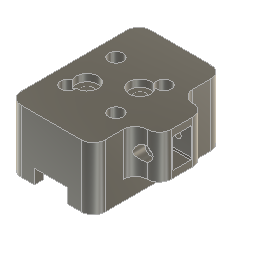
XY Bracket Bottom (Autodesk Fusion 360 archive; units mm, degrees)
design "XY Bracket Bottom Left"
part number: XY Brackets
part number: Left Bottom
Autodesk Fusion 360 part; units mm, degrees
sketch "Sketch1" plane through (0, 0, 0) normal (0, 0, 1) x (1, 0, 0) in component "Left Bottom"
  line L0 (27, -17.5) -> (-27, -17.5)
  line L1 (-27, -17.5) -> (-27, 17.5)
  line L2 (-27, 17.5) -> (27, 17.5)
  line L3 (27, 17.5) -> (27, -17.5)
  line L4 (27, -17.5) -> (-27, 17.5) construction
  line L5 (-27, -17.5) -> (27, 17.5) construction
  line L6 (23, 13.5) -> (-23, 13.5)
  line L7 (-23, 13.5) -> (-23, -13.5)
  line L8 (-23, -13.5) -> (23, -13.5)
  line L9 (23, -13.5) -> (23, 13.5)
  line L10 (23, 13.5) -> (-23, -13.5) construction
  line L11 (-23, 13.5) -> (23, -13.5) construction
  line L12 (27, 0) -> (23, 0) construction
  line L13 (-23, 0) -> (-27, 0) construction
  line L14 (23, -7) -> (27, -7)
  line L15 (27, -7) -> (27, 7)
  line L16 (27, 7) -> (23, 7)
  line L17 (23, 7) -> (23, -7)
  line L18 (23, -7) -> (27, 7) construction
  line L19 (27, -7) -> (23, 7) construction
  line L20 (-23, -7) -> (-27, -7)
  line L21 (-27, -7) -> (-27, 7)
  line L22 (-27, 7) -> (-23, 7)
  line L23 (-23, 7) -> (-23, -7)
  line L24 (-23, -7) -> (-27, 7) construction
  line L25 (-27, -7) -> (-23, 7) construction
  line L26 (10, -17.5) -> (10, 17.5) construction
  line L27 (-10, 17.5) -> (-10, -17.5) construction
  line L28 (27, -10) -> (-27, -10) construction
  line L29 (-27, 10) -> (27, 10) construction
  circle A0 centre (10, 10) radius 1.5
  circle A1 centre (10, 10) radius 3
  circle A2 centre (-10, 10) radius 1.5
  circle A3 centre (-10, 10) radius 3
  circle A4 centre (10, -10) radius 1.5
  circle A5 centre (10, -10) radius 3
  circle A6 centre (-10, -10) radius 1.5
  circle A7 centre (-10, -10) radius 3
  point P0 (25, 0)
  point P1 (-25, 0)
  dimension "d1" = 54
  dimension "d2" = 35
  dimension "d9" = 46
  dimension "d10" = 27
  dimension "d13" = 14
  dimension "d14" = 14
  dimension "d17" = 10
  dimension "d18" = 10
  dimension "d19" = 10
  dimension "d20" = 10
  dimension "d21" = 3
  dimension "d22" = 6
  dimension "d23" = 3
  dimension "d24" = 6
  dimension "d25" = 3
  dimension "d26" = 6
  dimension "d27" = 3
  dimension "d28" = 6
  constraint perpendicular L0 L1
  constraint parallel L0 L2
  constraint parallel L1 L3
  constraint horizontal L0
  constraint coincident L4 origin
  constraint coincident L5 origin
  constraint perpendicular L6 L7
  constraint parallel L6 L8
  constraint parallel L7 L9
  constraint horizontal L6
  constraint coincident L10 origin
  constraint coincident L11 origin
  constraint midpoint L3 L12.start
  constraint midpoint L9 L12.end
  constraint midpoint L7 L13.start
  constraint midpoint L1 L13.end
  constraint perpendicular L14 L15
  constraint parallel L14 L16
  constraint parallel L15 L17
  constraint horizontal L14
  constraint coincident L18 P0
  constraint coincident L19 P0
  constraint midpoint L12 P0
  constraint perpendicular L20 L21
  constraint parallel L20 L22
  constraint parallel L21 L23
  constraint horizontal L20
  constraint coincident L24 P1
  constraint coincident L25 P1
  constraint midpoint L13 P1
  constraint coincident L0 L26.start
  constraint coincident L2 L26.end
  constraint perpendicular L2 L26
  constraint coincident L2 L27.start
  constraint coincident L0 L27.end
  constraint perpendicular L0 L27
  constraint coincident L3 L28.start
  constraint coincident L1 L28.end
  constraint perpendicular L1 L28
  constraint coincident L1 L29.start
  constraint coincident L3 L29.end
  constraint perpendicular L3 L29
  constraint coincident L29 A0.centre
  constraint coincident L26 A0.centre
  constraint concentric A0 A1
  constraint coincident L27 A2.centre
  constraint coincident L29 A2.centre
  constraint concentric A2 A3
  constraint coincident L28 A4.centre
  constraint coincident L26 A4.centre
  constraint concentric A4 A5
  constraint coincident L27 A6.centre
  constraint coincident L28 A6.centre
  constraint concentric A6 A7
  measures "d1" distance of L1.end L2.end
  measures "d2" distance of L0.end L1.end
  measures "d9" distance of L7.end L8.end
  measures "d10" distance of L6.end L7.end
  measures "d13" distance of L14.end L15.end
  measures "d14" distance of L20.end L21.end
  measures "d17" distance of origin L26
  measures "d18" distance of origin L27
  measures "d19" distance of origin L28
  measures "d20" distance of origin L29
  measures "d21" diameter of A0
  measures "d22" diameter of A1
  measures "d23" diameter of A2
  measures "d24" diameter of A3
  measures "d25" diameter of A4
  measures "d26" diameter of A5
  measures "d27" diameter of A6
  measures "d28" diameter of A7
extrude "Extrude1" add sketch "Sketch1" along normal blind 26 contours L0 L1 L3 L7 L8 L9 L14 L20 | L3 L9 L14 L15 L16 L17 | L1 L7 L20 L21 L22 L23 | L1 L2 L3 L6 L7 L9 L16 L22 | L6 L7 L8 L9 L17 L23 | A0 | A1 | A2 | A3 | A4 | A5 | A6 | A7 in component "Left Bottom"
extrude "Extrude3" cut sketch "Sketch1" along normal blind 10 contours L6 L7 L8 L9 L17 L23 | A0 | A1 | A2 | A3 | A4 | A5 | A6 | A7 in component "Left Bottom"
extrude "Extrude4" cut sketch "Sketch1" along normal blind 6 contours L3 L9 L14 L15 L16 L17 | L1 L7 L20 L21 L22 L23 in component "Left Bottom"
extrude "Extrude6" cut sketch "Sketch1" along normal blind 13.8 contours A0 | A2 | A4 | A6 in component "Left Bottom"
extrude "Extrude7" cut sketch "Sketch1" along normal up to surface (12 mm away) from surface at 14 contours A0 | A1 | A2 | A3 | A4 | A5 | A6 | A7 in component "Left Bottom"
sketch "Sketch4" plane through (0, -17.5, 0) normal (0, -1, 0) x (1, 0, 0) in component "Left Bottom"
  line L0 (-27, 0) -> (27, 0)
  line L1 (27, 0) -> (27, 26)
  line L2 (27, 26) -> (-27, 26)
  line L3 (-27, 26) -> (-27, 0)
  line L4 (0, 26) -> (0, 0) construction
  line L5 (27, 17) -> (-27, 17) construction
  line L6 (9.5, 8) -> (-9.5, 8)
  line L7 (-9.5, 8) -> (-9.5, 26)
  line L8 (-9.5, 26) -> (9.5, 26)
  line L9 (9.5, 26) -> (9.5, 8)
  line L10 (9.5, 8) -> (-9.5, 26) construction
  line L11 (-9.5, 8) -> (9.5, 26) construction
  line L12 (6.125, 14.5697) -> (6.125, 11.5619) construction
  line L13 (5.3053, 13.75) -> (8.1776, 13.75) construction
  line L14 (-6.125, 21.5015) -> (-6.125, 24.7576) construction
  line L15 (-5.6265, 22) -> (-10.4628, 22) construction
  line L16 (5.4553, 22) -> (9.3664, 22) construction
  line L17 (6.125, 21.3303) -> (6.125, 24.7948) construction
  line L18 (5.4553, 22) -> (8.9906, 22) construction
  line L19 (4.125, 10.875) -> (-4.125, 10.875)
  line L20 (-4.125, 10.875) -> (-4.125, 23.125)
  line L21 (-4.125, 23.125) -> (4.125, 23.125)
  line L22 (4.125, 23.125) -> (4.125, 10.875)
  line L23 (4.125, 10.875) -> (-4.125, 23.125) construction
  line L24 (-4.125, 10.875) -> (4.125, 23.125) construction
  line L25 (-4.125, 22.625) -> (4.125, 22.625) construction
  line L26 (3.625, 23.125) -> (3.625, 10.875) construction
  line L27 (4.125, 11.375) -> (-4.125, 11.375) construction
  line L28 (-3.625, 10.875) -> (-3.625, 23.125) construction
  line L29 (-3.625, 10.875) -> (-4.125, 11.375)
  line L30 (-4.125, 22.625) -> (-3.625, 23.125)
  line L31 (3.625, 23.125) -> (4.125, 22.625)
  line L32 (4.125, 11.375) -> (3.625, 10.875)
  dimension "d47" = 9
  dimension "d48" = 19
  dimension "d49" = 18
  dimension "d93" = 12.25
  dimension "d94" = 8.25
  dimension "d95" = 0.5
  dimension "d96" = 0.5
  dimension "d97" = 0.5
  dimension "d98" = 0.5
  dimension "d104" = 17.5
  constraint midpoint L2 L4.start
  constraint coincident L4.end origin
  constraint coincident L1 L5.start
  constraint coincident L3 L5.end
  constraint perpendicular L3 L5
  constraint perpendicular L6 L7
  constraint parallel L6 L8
  constraint parallel L7 L9
  constraint horizontal L6
  constraint perpendicular L12 L13
  constraint coincident L16 L18.end
  constraint perpendicular L19 L20
  constraint parallel L19 L21
  constraint horizontal L19
  constraint coincident L20 L25.start
  constraint coincident L22 L25.end
  constraint perpendicular L22 L25
  constraint coincident L21 L26.start
  constraint coincident L19 L26.end
  constraint perpendicular L19 L26
  constraint coincident L22 L27.start
  constraint coincident L20 L27.end
  constraint perpendicular L20 L27
  constraint coincident L19 L28.start
  constraint coincident L21 L28.end
  constraint perpendicular L21 L28
  measures "d47" distance of L2 L5
  measures "d48" distance of L7.end L8.end
  measures "d49" distance of L6.end L7.end
  measures "d93" distance of L19.end L20.end
  measures "d94" distance of L20.end L21.end
  measures "d95" distance of L20 L28
  measures "d96" distance of L21 L25
  measures "d97" distance of L22 L26
  measures "d98" distance of L19 L27
  measures "d104" distance of L3 L7
extrude "Extrude9" add sketch "Sketch4" along normal blind 10 contours L2 L6 L7 L8 L9 | L19 L22 L32 | L19 L20 L21 L22 L29 L30 L31 L32 | L19 L20 L29 | L21 L22 L31 | L20 L21 L30 in component "Left Bottom"
extrude "Extrude10" cut sketch "Sketch4" against normal blind 17.5 from surface at 10 contours L19 L20 L21 L22 L29 L30 L31 L32 in component "Left Bottom"
sketch "Sketch5" plane through (-9.5, 0, 0) normal (-1, 0, 0) x (0, -1, 0) in component "Left Bottom"
  line L0 (17.5, 26) -> (17.5, 8)
  line L1 (17.5, 8) -> (27.5, 8)
  line L2 (27.5, 8) -> (27.5, 26)
  line L3 (27.5, 26) -> (17.5, 26)
  line L4 (21.5, 20.1754) -> (18.75, 18.5877)
  line L5 (18.75, 18.5877) -> (18.75, 15.4123)
  line L6 (18.75, 15.4123) -> (21.5, 13.8246)
  line L7 (21.5, 13.8246) -> (24.25, 15.4123)
  line L8 (24.25, 15.4123) -> (24.25, 18.5877)
  line L9 (24.25, 18.5877) -> (21.5, 20.1754)
  circle A0 centre (21.5, 17) radius 3
  circle A1 centre (21.5, 17) radius 1.5
  line L10 (17.5, 8) -> (17.5, 26)
  point P0 (21.5, 17)
  dimension "d99" = 2.75
  dimension "d100" = 6
  dimension "d101" = 3
  dimension "d103" = 4
  dimension "d114" = 9
  constraint coincident P0 A0.centre
  constraint parallel L2 L8
  measures "d99" distance of P0 L9
  measures "d100" diameter of A0
  measures "d101" diameter of A1
  measures "d103" distance of P0 L10
  measures "d114" distance of L3 P0
extrude "Extrude17" cut sketch "Sketch5" along normal blind 3 from surface at -19 contours L4 L9 A0 | L4 L5 L6 L7 L8 L9 A0 | L4 L5 A0 | L8 L9 A0 | L5 L6 A0 | L7 L8 A0 | L6 L7 A0 in component "Left Bottom"
extrude "Extrude18" cut sketch "Sketch5" against normal up to surface (19 mm away) contours A1 in component "Left Bottom"
extrude "Extrude19" cut sketch "Sketch5" against normal blind 3 contours L4 L5 L6 L7 L8 L9 A0 | L4 A0 | L9 A0 | L5 A0 | L8 A0 | L6 A0 | L7 A0 in component "Left Bottom"
sketch "Sketch3" plane through (0, 0, 26) normal (0, 0, 1) x (-1, 0, 0) in component "Left Bottom"
  line L0 (-27, -17.5) -> (27, -17.5)
  line L1 (27, -17.5) -> (27, 17.5)
  line L2 (27, 17.5) -> (9.5, 17.5)
  line L3 (-27, 17.5) -> (-27, -17.5)
  line L4 (-14.5, 16.5) -> (14.5, 16.5)
  line L5 (14.5, 16.5) -> (14.5, -16.5)
  line L6 (14.5, -16.5) -> (-14.5, -16.5)
  line L7 (-14.5, -16.5) -> (-14.5, 16.5)
  line L8 (-14.5, 16.5) -> (14.5, -16.5) construction
  line L9 (14.5, 16.5) -> (-14.5, -16.5) construction
  line L10 (-4, -16.5) -> (-4, 16.5) construction
  line L11 (-14.5, 6) -> (14.5, 6) construction
  line L12 (14.5, -7) -> (-14.5, -7) construction
  line L13 (5, -16.5) -> (5, 16.5) construction
  circle A0 centre (5, -7) radius 2.5
  circle A1 centre (-4, 6) radius 2.5
  line L14 (9.5, 17.5) -> (9.5, 27.5)
  line L15 (9.5, 27.5) -> (-9.5, 27.5)
  line L16 (-9.5, 27.5) -> (-9.5, 17.5)
  line L17 (-9.5, 17.5) -> (-27, 17.5)
  line L18 (-9.5, 17.5) -> (-11.4807, 17.5) construction
  line L19 (-11.4807, 17.5) -> (9.5, 17.5) construction
  line L20 (-9.5, 21.5) -> (9.5, 21.5) construction
  line L21 (2.5, 17.5) -> (2.5, 27.5) construction
  circle A2 centre (0, 21.5) radius 1.5
  circle A3 centre (0, 21.5) radius 3
  line L22 (-1.5877, 18.75) -> (1.5877, 18.75)
  line L23 (1.5877, 18.75) -> (3.1754, 21.5)
  line L24 (3.1754, 21.5) -> (1.5877, 24.25)
  line L25 (1.5877, 24.25) -> (-1.5877, 24.25)
  line L26 (-1.5877, 24.25) -> (-3.1754, 21.5)
  line L27 (-3.1754, 21.5) -> (-1.5877, 18.75)
  circle A4 centre (-4, 6) radius 4.5
  circle A5 centre (5, -7) radius 4.5
  circle A6 centre (-10, -10) radius 3
  circle A7 centre (10, 10) radius 3
  circle A8 centre (10, -10) radius 3
  circle A9 centre (-10, 10) radius 3
  line L28 (7.3094, -3) -> (2.6906, -3)
  line L29 (2.6906, -3) -> (0.3812, -7)
  line L30 (0.3812, -7) -> (2.6906, -11)
  line L31 (2.6906, -11) -> (7.3094, -11)
  line L32 (7.3094, -11) -> (9.6188, -7)
  line L33 (9.6188, -7) -> (7.3094, -3)
  line L34 (0.6188, 6) -> (-1.6906, 10)
  line L35 (-1.6906, 10) -> (-6.3094, 10)
  line L36 (-6.3094, 10) -> (-8.6188, 6)
  line L37 (-8.6188, 6) -> (-6.3094, 2)
  line L38 (-6.3094, 2) -> (-1.6906, 2)
  line L39 (-1.6906, 2) -> (0.6188, 6)
  point P0 (0, 21.5)
  point P1 (5, -7)
  point P2 (-4, 6)
  dimension "d29" = 29
  dimension "d30" = 33
  dimension "d38" = 10.5
  dimension "d39" = 9.5
  dimension "d40" = 9.5
  dimension "d41" = 10.5
  dimension "d42" = 5
  dimension "d43" = 5
  dimension "d56" = 4
  dimension "d58" = 12
  dimension "d59" = 3
  dimension "d60" = 6
  dimension "d61" = 2.75
  dimension "d71" = 9
  dimension "d72" = 9
  dimension "d85" = 4
  dimension "d86" = 4
  constraint perpendicular L4 L5
  constraint parallel L4 L6
  constraint parallel L5 L7
  constraint horizontal L4
  constraint coincident L8 origin
  constraint coincident L9 origin
  constraint coincident L6 L10.start
  constraint coincident L4 L10.end
  constraint perpendicular L4 L10
  constraint coincident L7 L11.start
  constraint coincident L5 L11.end
  constraint perpendicular L5 L11
  constraint coincident L5 L12.start
  constraint coincident L7 L12.end
  constraint perpendicular L7 L12
  constraint coincident L6 L13.start
  constraint coincident L4 L13.end
  constraint perpendicular L4 L13
  constraint coincident L13 P1
  constraint coincident L12 P1
  constraint coincident L10 P2
  constraint coincident L11 P2
  constraint coincident L16.end L17.start
  constraint coincident L2.end L14.start
  constraint perpendicular L14 L19
  constraint coincident L16 L20.start
  constraint coincident L14 L20.end
  constraint perpendicular L14 L20
  constraint coincident L19 L21.start
  constraint coincident L15 L21.end
  constraint perpendicular L15 L21
  constraint midpoint L20 P0
  constraint concentric A2 A3
  constraint coincident P0 A2.centre
  constraint parallel L19 L22
  constraint concentric A1 A4
  constraint concentric A0 A5
  constraint coincident P1 A0.centre
  constraint coincident P2 A1.centre
  constraint parallel L4 L35
  constraint parallel L6 L31
  measures "d29" distance of L5.end L6.end
  measures "d30" distance of L4.end L5.end
  measures "d38" distance of L4 L11
  measures "d39" distance of L5 L13
  measures "d40" distance of L6 L12
  measures "d41" distance of L7 L10
  measures "d42" diameter of A0
  measures "d43" diameter of A1
  measures "d56" distance of L19 L20
  measures "d58" distance of L16 L21
  measures "d59" diameter of A2
  measures "d60" diameter of A3
  measures "d61" distance of P0 L27
  measures "d71" diameter of A4
  measures "d72" diameter of A5
  measures "d85" distance of P1 L33
  measures "d86" distance of P2 L39
extrude "Extrude8" cut sketch "Sketch3" against normal blind 10 from surface at -3.2 contours A0 | A1 in component "Left Bottom"
extrude "Extrude14" cut sketch "Sketch3" against normal blind 3 contours A0 | A1 | A4 L34 L35 L36 L37 L38 L39 | A4 L34 | A4 L39 | A4 L35 | A4 L38 | A4 A9 L36 | A4 L37 | A4 A9 | A5 A8 L28 L29 L30 L31 L33 | A5 L33 | A5 A8 L32 | A5 L32 | A5 L28 | A5 L31 | A5 L29 | A5 L30 picked at (-7.7899, 8.241) picked at (8.2012, -8.7013) in component "Left Bottom"
extrude "Extrude16" cut sketch "Sketch3" against normal up to surface (8 mm away) from surface at -8 contours A0 | A1 | A4 L34 L35 L36 L37 L38 L39 | A5 A8 L28 L29 L30 L31 L33 | A5 A8 L32 picked at (8.2012, -8.7013) in component "Left Bottom"
fillet "Fillet2" radius 5 8 edges at (27, -17.5, 13) (27, 17.5, 13) (-27, 17.5, 13) (-27, -17.5, 13) (9.5, -17.5, 17) (-9.5, -17.5, 17) (-9.5, -27.5, 17) (9.5, -27.5, 17) in component "Left Bottom"
component "Left Bottom" placed x (-0.000001, 1, 0) y (-1, -0.000001, 0) z (0, 0, 1) at (0, 0, 0)
